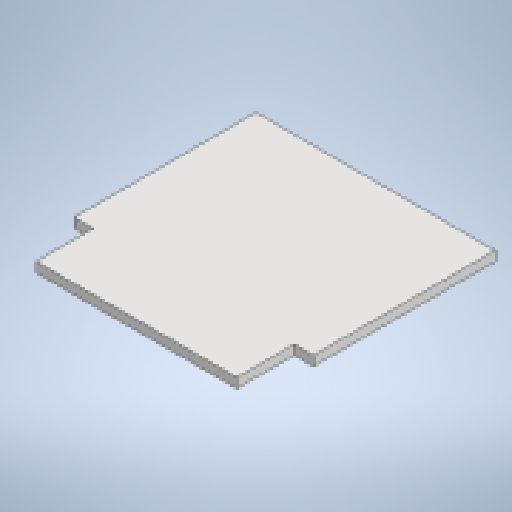
# Autodesk Inventor part: spod
Saved by Autodesk Inventor 2023 (Build 270158000, 158)
## iProperties
Created: 2023-07-30
Part Number: spod
Material: Stal, węglowa
Document SubType Name: Modeling
Designer: Kamil
Density: 7.85 g/cm^3
Appearance: Częściowo polerowany
Author: Kamil
Autodesk Inventor part; units mm, degrees
ref_plane "YZ Plane" through (0, 0, 0) normal (1, 0, 0) x (0, 1, 0)
ref_plane "XZ Plane" through (0, 0, 0) normal (0, 1, 0) x (-1, 0, 0)
ref_plane "XY Plane" through (0, 0, 0) normal (0, 0, 1) x (1, 0, 0)
sketch "Szkic1" plane through (0, 0, 0) normal (0, 1, 0) x (-1, 0, 0)
  line L0 (0, 0) -> (50, 0)
  line L1 (50, 0) -> (50, -50)
  line L2 (50, -50) -> (0, -50)
  line L3 (0, -50) -> (0, 0)
  dimension "d0" = 50
  dimension "d1" = 50
  constraints: 8 end point, 2 parallel, 1 horizontal, 1 perpendicular
  measures "d0" distance of L1.end L2.end
  measures "d1" distance of L0.end L1.end
extrude "Wyciągnięcie proste1" add sketch "Szkic1" along normal blind 2
sketch "Szkic2" plane through (0, 2, 0) normal (0, 1, 0) x (1, 0, 0)
  line L0 (0, 50) -> (-50, 50) projected
  line L1 (-50, 50) -> (-50, 0) projected
  line L2 (-50, 0) -> (0, 0) projected
  line L3 (0, 0) -> (0, 50) projected
  line L4 (0, 0) -> (-14, 0)
  line L5 (-14, 0) -> (-14, 14)
  line L6 (-14, 14) -> (0, 14)
  line L7 (0, 14) -> (0, 0)
  line L8 (-50, 0) -> (-36, 0)
  line L9 (-36, 0) -> (-36, 14)
  line L10 (-36, 14) -> (-50, 14)
  line L11 (-50, 14) -> (-50, 0)
  point P0 (-36, 0)
  point P1 (0, 14)
  point P2 (-14, 0)
  dimension "d4" = 14
  dimension "d5" = 14
  dimension "d8" = 14
  dimension "d11" = 14
  constraints: 16 end point, 4 parallel, 2 horizontal, 2 perpendicular, 1 point on line
  measures "d4" distance of L5.end L6.end
  measures "d5" distance of L4.end L5.end
  measures "d8" distance of L8.end L9.end
  measures "d11" distance of L9.end L10.end
extrude "Wyciągnięcie proste2" cut sketch "Szkic2" against normal through all contours L3 L2 L5 L6 | L10 L9 L2 L1
sketch "Szkic3" plane through (-50, 0, -50) normal (-1, 0, 0) x (0, 0, 1)
  line L0 (48.0005, -17) -> (8.7747, -17) projected
  line L1 (8.7747, -17) -> (2.0995, 3.9) projected
  line L2 (2.0995, 3.9) -> (0, 3.9) projected
  line L3 (0, 3.9) -> (7.3139, -19) projected
  line L4 (7.3139, -19) -> (50.0005, -19) projected
  line L5 (50.0005, -19) -> (50.0005, -17) projected
  line L6 (50.0005, -17) -> (50, -17) projected
  line L7 (50, -17) -> (50, 0) projected
  line L8 (50, 0) -> (48.0005, 0) projected
  line L9 (48.0005, 0) -> (48.0005, -17) projected
  line L10 (36, 0) -> (36, 2) projected
  line L11 (0, 2) -> (36, 2) projected
  line L12 (0, 0) -> (0, 2) projected
  line L13 (0, 0) -> (36, 0) projected
  point P0 (3.3451, 0)
  point P1 (2.7064, 2)
extrude "Wyciągnięcie proste3" cut sketch "Szkic3" against normal through all contours L13 L3 L11 L1 | L13 L12 L11 L3
